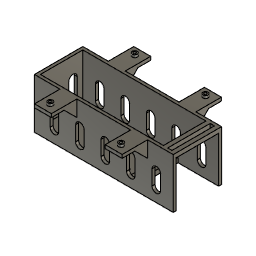
Battery Housing Vertical Slits (Autodesk Fusion 360 design; units mm, degrees)
Autodesk Fusion 360 part; units mm, degrees
sketch "Sketch1" plane through (0, 0, 0) normal (1, 0, 0) x (0, 1, 0)
  line L0 (0, 0) -> (57, 0)
  line L1 (57, 0) -> (57, 57)
  line L2 (57, 57) -> (0, 57)
  line L3 (0, 57) -> (0, 0)
  line L4 (3.5, 57) -> (53.5, 57)
  line L5 (53.5, 57) -> (53.5, 3.5)
  line L6 (53.5, 3.5) -> (3.5, 3.5)
  line L7 (3.5, 3.5) -> (3.5, 57)
  dimension "d1" = 57
  dimension "d2" = 57
  dimension "d3" = 3.5
  dimension "d4" = 3.5
  dimension "d5" = 3.5
  constraint horizontal L0
  constraint vertical L1
  constraint horizontal L2
  constraint vertical L3
  constraint coincident L0.start L3.end
  constraint horizontal L4
  constraint vertical L5
  constraint horizontal L6
  constraint vertical L7
  constraint coincident L2 L4.start
  measures "d1" distance of L0.start L0.end
  measures "d2" distance of L0.start L2.end
  measures "d3" distance of L1 L5
  measures "d4" distance of L3 L7
  measures "d5" distance of L0 L6
extrude "Extrude1" add sketch "Sketch1" along normal blind 160 contours L0 L1 L2 L3 L5 L6 L7
sketch "Sketch2" plane through (0, 0, 0) normal (-1, 0, 0) x (0, -1, 0)
  line L0 (-3.5, 57) -> (-3.5, 3.5)
  line L1 (-3.5, 3.5) -> (-53.5, 3.5)
  line L2 (-53.5, 3.5) -> (-53.5, 57)
  line L3 (-53.5, 57) -> (-57, 57)
  line L4 (-57, 57) -> (-57, 0)
  line L5 (-57, 0) -> (0, 0)
  line L6 (0, 0) -> (0, 57)
  line L7 (0, 57) -> (-3.5, 57)
  line L8 (-57, 57) -> (0, 57)
  line L9 (0, 57) -> (0, 0)
  line L10 (0, 0) -> (-57, 0)
  line L11 (-57, 0) -> (-57, 57)
  constraint horizontal L8
  constraint vertical L9
  constraint horizontal L10
  constraint vertical L11
  constraint coincident L5.end L6.start
  constraint coincident L3.end L4.start
extrude "Extrude2" add sketch "Sketch2" along normal blind 3.5
ref_plane "WorkPlane1" through (78.25, 28.5, 57) normal (0, 0, 1) x (0, -1, 0)
sketch "Sketch4" plane through (0, 0, 57) normal (0, 0, 1) x (1, 0, 0)
  circle A0 centre (36.5, 78.25) radius 1.5
  circle A1 centre (119.8, 78.25) radius 1.5
  circle A2 centre (36.5, -21.25) radius 1.5
  circle A3 centre (119.8, -21.25) radius 1.5
  line L0 (-3.5, 57) -> (160, 57)
  line L1 (26.5, 0) -> (46.5, 0)
  line L2 (46.5, 0) -> (46.5, -30)
  line L3 (46.5, -30) -> (26.5, -30)
  line L4 (26.5, -30) -> (26.5, 0)
  line L5 (109.8, 0) -> (129.8, 0)
  line L6 (129.8, 0) -> (129.8, -30)
  line L7 (129.8, -30) -> (109.8, -30)
  line L8 (109.8, -30) -> (109.8, 0)
  line L9 (109.8, 57) -> (129.8, 57)
  line L10 (129.8, 57) -> (129.8, 87)
  line L11 (129.8, 87) -> (109.8, 87)
  line L12 (109.8, 87) -> (109.8, 57)
  line L13 (26.5, 87) -> (46.5, 87)
  line L14 (46.5, 87) -> (46.5, 57)
  line L15 (46.5, 57) -> (26.5, 57)
  line L16 (26.5, 57) -> (26.5, 87)
  line L17 (-3.5, 57) -> (-3.5, 54.574)
  line L18 (-3.5, 0) -> (-3.5, 57)
  point P0 (-3.5, 57)
  dimension "d27" = 3
  dimension "d29" = 3
  dimension "d31" = 3
  dimension "d33" = 3
  dimension "d38" = 21.25
  dimension "d39" = 10
  dimension "d40" = 10
  dimension "d41" = 20
  dimension "d42" = 30
  dimension "d43" = 20
  dimension "d44" = 30
  dimension "d45" = 10
  dimension "d46" = 10
  dimension "d47" = 21.25
  dimension "d51" = 30
  dimension "d52" = 20
  dimension "d53" = 30
  dimension "d54" = 20
  dimension "d186" = 63.3
  dimension "d187" = 63.3
  dimension "d188" = 103.3
  dimension "d189" = 163.5
  dimension "d190" = 30
  dimension "d191" = 30
  constraint horizontal L1
  constraint vertical L2
  constraint horizontal L3
  constraint vertical L4
  constraint horizontal L5
  constraint vertical L6
  constraint horizontal L7
  constraint vertical L8
  constraint horizontal L9
  constraint vertical L10
  constraint horizontal L11
  constraint vertical L12
  constraint horizontal L13
  constraint vertical L14
  constraint horizontal L15
  constraint vertical L16
  constraint coincident P0 L0.start
  constraint perpendicular L0 L17
  measures "d27" diameter of A0
  measures "d29" diameter of A1
  measures "d31" diameter of A2
  measures "d33" diameter of A3
  measures "d38" distance of A0.centre L0
  measures "d39" distance of A3.centre L8
  measures "d40" distance of A2.centre L4
  measures "d41" distance of L9.start L9.end
  measures "d42" distance of L9.start L11.end
  measures "d43" distance of L13.start L13.end
  measures "d44" distance of L13.start L15.end
  measures "d45" distance of A1.centre L12
  measures "d46" distance of A0.centre L16
  measures "d47" distance of A0.centre L15
  measures "d51" distance of L5.end L6.end
  measures "d52" distance of L6.end L7.end
  measures "d53" distance of L1.end L2.end
  measures "d54" distance of L2.end L3.end
  measures "d186" distance of L12 L14
  measures "d187" distance of L2 L8
  measures "d188" distance of L10 L16
  measures "d189" distance of P0 L0.end
  measures "d190" distance of L16 L18
  measures "d191" distance of L4 L18
extrude "Extrude4" add sketch "Sketch4" against normal blind 4
sketch "Sketch5" plane through (129.8, 0, 0) normal (1, 0, 0) x (0, 1, 0)
  line L0 (0, 57) -> (-30, 57)
  line L1 (-30, 57) -> (-30, 53)
  line L2 (-30, 53) -> (0, 53)
  line L3 (0, 53) -> (0, 57)
  line L4 (0, 53) -> (-15, 53)
  line L5 (-15, 53) -> (0, 38)
  line L6 (0, 38) -> (0, 53)
  dimension "d55" = 45
  constraint coincident L2.end L3.start
  constraint midpoint L2 L4.end
  constraint perpendicular L4 L6
  measures "d55" angle of L4 L5
extrude "Extrude5" add sketch "Sketch5" against normal blind 2 contours L2 L4 L5 L6
sketch "Sketch6" plane through (129.8, 0, 0) normal (1, 0, 0) x (0, 1, 0)
  line L0 (87, 57) -> (57, 57)
  line L1 (57, 57) -> (57, 53)
  line L2 (57, 53) -> (87, 53)
  line L3 (87, 53) -> (87, 57)
  line L4 (57, 53) -> (72, 53)
  line L5 (72, 53) -> (57, 38)
  line L6 (57, 38) -> (57, 53)
  dimension "d58" = 45
  constraint coincident L1.end L2.start
  constraint midpoint L2 L4.end
  constraint perpendicular L2 L6
  measures "d58" angle of L4 L5
extrude "Extrude6" add sketch "Sketch6" against normal blind 2 contours L2 L4 L5 L6
sketch "Sketch7" plane through (109.8, 0, 0) normal (-1, 0, 0) x (0, -1, 0)
  line L0 (-57, 57) -> (-87, 57)
  line L1 (-87, 57) -> (-87, 53)
  line L2 (-87, 53) -> (-57, 53)
  line L3 (-57, 53) -> (-57, 57)
  line L4 (-57, 53) -> (-72, 53)
  line L5 (-72, 53) -> (-57, 38)
  line L6 (-57, 38) -> (-57, 53)
  dimension "d61" = 45
  constraint coincident L2.end L3.start
  constraint midpoint L2 L4.end
  constraint perpendicular L4 L6
  measures "d61" angle of L4 L5
extrude "Extrude7" add sketch "Sketch7" against normal blind 2 contours L2 L4 L5 L6
sketch "Sketch8" plane through (109.8, 0, 0) normal (-1, 0, 0) x (0, -1, 0)
  line L0 (30, 57) -> (0, 57)
  line L1 (0, 57) -> (0, 53)
  line L2 (0, 53) -> (30, 53)
  line L3 (30, 53) -> (30, 57)
  line L4 (0, 53) -> (15, 53)
  line L5 (15, 53) -> (0, 38)
  line L6 (0, 38) -> (0, 53)
  dimension "d64" = 45
  constraint coincident L1.end L2.start
  constraint midpoint L2 L4.end
  constraint perpendicular L4 L6
  measures "d64" angle of L4 L5
extrude "Extrude8" add sketch "Sketch8" against normal blind 2 contours L2 L4 L5 L6
sketch "Sketch9" plane through (46.5, 0, 0) normal (1, 0, 0) x (0, 1, 0)
  line L0 (0, 57) -> (-30, 57)
  line L1 (-30, 57) -> (-30, 53)
  line L2 (-30, 53) -> (0, 53)
  line L3 (0, 53) -> (0, 57)
  line L4 (0, 53) -> (-15, 53)
  line L5 (-15, 53) -> (0, 38)
  line L6 (0, 38) -> (0, 53)
  dimension "d67" = 45
  constraint coincident L2.end L3.start
  constraint midpoint L2 L4.end
  constraint perpendicular L4 L6
  measures "d67" angle of L4 L5
extrude "Extrude9" add sketch "Sketch9" against normal blind 2 contours L2 L4 L5 L6
sketch "Sketch10" plane through (26.5, 0, 0) normal (-1, 0, 0) x (0, -1, 0)
  line L0 (30, 57) -> (0, 57)
  line L1 (0, 57) -> (0, 53)
  line L2 (0, 53) -> (30, 53)
  line L3 (30, 53) -> (30, 57)
  line L4 (0, 53) -> (15, 53)
  line L5 (15, 53) -> (0, 38)
  line L6 (0, 38) -> (0, 53)
  constraint coincident L1.end L2.start
  constraint midpoint L2 L4.end
  constraint perpendicular L4 L6
extrude "Extrude10" add sketch "Sketch10" against normal blind 2 contours L2 L4 L5 L6
sketch "Sketch11" plane through (26.5, 0, 0) normal (-1, 0, 0) x (0, -1, 0)
  line L0 (-57, 57) -> (-87, 57)
  line L1 (-87, 57) -> (-87, 53)
  line L2 (-87, 53) -> (-57, 53)
  line L3 (-57, 53) -> (-57, 57)
  line L4 (-57, 53) -> (-72, 53)
  line L5 (-72, 53) -> (-57, 38)
  line L6 (-57, 38) -> (-57, 53)
  constraint coincident L2.end L3.start
  constraint midpoint L2 L4.end
extrude "Extrude11" add sketch "Sketch11" against normal blind 2 contours L2 L4 L5 L6
sketch "Sketch12" plane through (46.5, 0, 0) normal (1, 0, 0) x (0, 1, 0)
  line L0 (87, 57) -> (57, 57)
  line L1 (57, 57) -> (57, 53)
  line L2 (57, 53) -> (87, 53)
  line L3 (87, 53) -> (87, 57)
  line L4 (57, 53) -> (72, 53)
  line L5 (72, 53) -> (57, 38)
  line L6 (57, 38) -> (57, 53)
  dimension "d74" = 45
  constraint coincident L1.end L2.start
  constraint midpoint L2 L4.end
  constraint perpendicular L4 L6
  measures "d74" angle of L4 L5
extrude "Extrude12" add sketch "Sketch12" against normal blind 2 contours L2 L4 L5 L6
extrude "Extrude20" add 1 faces at (105.5, 38, 0) along direction (0, 0, -1) blind 2
sketch "Sketch23" plane through (0, 0, 3.5) normal (0, 0, 1) x (-1, 0, 0)
  line L0 (0, -53.5) -> (0, -3.5)
  line L1 (0, -3.5) -> (-160, -3.5)
  line L2 (-160, -3.5) -> (-160, -53.5)
  line L3 (-160, -53.5) -> (0, -53.5)
  line L4 (-160, -53.5) -> (-102.25, -53.5)
  line L5 (-102.25, -53.5) -> (-102.25, -3.5)
  line L6 (-102.25, -3.5) -> (-160, -3.5)
  line L7 (-160, -3.5) -> (-160, -53.5)
  constraint horizontal L4
  constraint vertical L5
  constraint horizontal L6
  constraint vertical L7
  constraint coincident L1 L5.end
  constraint coincident L2.end L3.start
extrude "Extrude22" cut sketch "Sketch23" against normal up to surface (5.5 mm away) contours L1 L2 L3 L4 L5 L6 L7
sketch "Sketch28" plane through (0, 0, 57) normal (0, 0, 1) x (-1, 0, 0)
  line L0 (-160, 0) -> (-160, -3.5)
  line L1 (-160, -57) -> (-129.8, -57)
  line L2 (-129.8, -57) -> (-129.8, -87)
  line L3 (-129.8, -87) -> (-109.8, -87)
  line L4 (-109.8, -87) -> (-109.8, -57)
  line L5 (-109.8, -57) -> (-46.5, -57)
  line L6 (-46.5, -57) -> (-46.5, -87)
  line L7 (-46.5, -87) -> (-26.5, -87)
  line L8 (-26.5, -87) -> (-26.5, -57)
  line L9 (-26.5, -57) -> (3.5, -57)
  line L10 (3.5, -57) -> (3.5, 0)
  line L11 (3.5, 0) -> (-26.5, 0)
  line L12 (-26.5, 0) -> (-26.5, 30)
  line L13 (-26.5, 30) -> (-46.5, 30)
  line L14 (-46.5, 30) -> (-46.5, 0)
  line L15 (-46.5, 0) -> (-109.8, 0)
  line L16 (-109.8, 0) -> (-109.8, 30)
  line L17 (-109.8, 30) -> (-129.8, 30)
  line L18 (-129.8, 30) -> (-129.8, 0)
  line L19 (-129.8, 0) -> (-160, 0)
  line L20 (0, -3.5) -> (0, -53.5)
  line L21 (0, -53.5) -> (-160, -53.5)
  line L22 (-160, -3.5) -> (0, -3.5)
  circle A0 centre (-119.8, 21.25) radius 1.5
  circle A1 centre (-36.5, 21.25) radius 1.5
  circle A2 centre (-119.8, -78.25) radius 1.5
  circle A3 centre (-36.5, -78.25) radius 1.5
  circle A4 centre (-36.5, -78.25) radius 1.5
  circle A5 centre (-119.8, -78.25) radius 1.5
  circle A6 centre (-36.5, 21.25) radius 1.5
  circle A7 centre (-119.8, 21.25) radius 1.5
  circle A8 centre (-119.8, 21.25) radius 3
  circle A9 centre (-36.5, 21.25) radius 3
  circle A10 centre (-36.5, -78.25) radius 3
  circle A11 centre (-119.8, -78.25) radius 3
  line L23 (-160, -53.5) -> (-160, -57)
  dimension "d249" = 3
  dimension "d250" = 3
  dimension "d251" = 3
  dimension "d252" = 3
  dimension "d253" = 6
  dimension "d254" = 6
  dimension "d255" = 6
  dimension "d256" = 6
  constraint concentric A3 A4
  constraint concentric A2 A5
  constraint concentric A1 A6
  constraint concentric A0 A7
  constraint concentric A0 A8
  constraint concentric A6 A9
  constraint concentric A4 A10
  constraint concentric A5 A11
  measures "d249" diameter of A4
  measures "d250" diameter of A5
  measures "d251" diameter of A6
  measures "d252" diameter of A7
  measures "d253" diameter of A8
  measures "d254" diameter of A9
  measures "d255" diameter of A10
  measures "d256" diameter of A11
extrude "Extrude27" add sketch "Sketch28" along normal blind 3 contours A8 | A9 | A10 | A11
sketch "Sketch30" plane through (0, 57, 0) normal (0, 1, 0) x (-1, 0, 0)
  line L0 (-46.5, 38) -> (-46.5, 57)
  line L1 (-46.5, 57) -> (-109.8, 57)
  line L2 (-109.8, 57) -> (-109.8, 38)
  line L3 (-109.8, 38) -> (-111.8, 38)
  line L4 (-111.8, 38) -> (-111.8, 53)
  line L5 (-111.8, 53) -> (-127.8, 53)
  line L6 (-127.8, 53) -> (-127.8, 38)
  line L7 (-127.8, 38) -> (-129.8, 38)
  line L8 (-129.8, 38) -> (-129.8, 57)
  line L9 (-129.8, 57) -> (-160, 57)
  line L10 (-160, 57) -> (-160, -2)
  line L11 (-160, -2) -> (3.5, -2)
  line L12 (3.5, -2) -> (3.5, 57)
  line L13 (3.5, 57) -> (-26.5, 57)
  line L14 (-26.5, 57) -> (-26.5, 38)
  line L15 (-26.5, 38) -> (-28.5, 38)
  line L16 (-28.5, 38) -> (-28.5, 53)
  line L17 (-28.5, 53) -> (-44.5, 53)
  line L18 (-44.5, 53) -> (-44.5, 38)
  line L19 (-44.5, 38) -> (-46.5, 38)
  arc A0 (-140, 35) -> (-140, 25) centre (-140, 30) ccw
  arc A1 (-140, 17.5) -> (-140, 7.5) centre (-140, 12.5) ccw
  line L20 (-140, 30) -> (-110, 30)
  line L21 (-105, 30) -> (-85, 30)
  line L22 (-80, 30) -> (-55, 30)
  line L23 (-50, 30) -> (-20, 30)
  line L24 (-140, 12.5) -> (-110, 12.5)
  line L25 (-105, 12.5) -> (-80, 12.5)
  line L26 (-75, 12.5) -> (-55, 12.5)
  line L27 (-145, 30) -> (-145, 12.5)
  line L28 (-135, 30) -> (-135, 12.5)
  line L29 (-115, 30) -> (-115, 12.5)
  line L30 (-105, 30) -> (-105, 12.5)
  line L31 (-75, 30) -> (-75, 12.5)
  line L32 (-85, 30) -> (-85, 12.5)
  line L33 (-45, 30) -> (-45, 12.5)
  line L34 (-55, 30) -> (-55, 12.5)
  line L35 (-25, 30) -> (-25, 12.5)
  line L36 (-15, 30) -> (-15, 12.5)
  arc A2 (-25, 12.5) -> (-15, 12.5) centre (-20, 12.5) ccw
  arc A3 (-15, 30) -> (-25, 30) centre (-20, 30) ccw
  arc A4 (-55, 12.5) -> (-45, 12.5) centre (-50, 12.5) ccw
  arc A5 (-45, 30) -> (-55, 30) centre (-50, 30) ccw
  line L37 (-75, 12.5) -> (-20, 12.5)
  arc A6 (-85, 12.5) -> (-75, 12.5) centre (-80, 12.5) ccw
  arc A7 (-75, 30) -> (-85, 30) centre (-80, 30) ccw
  arc A8 (-105, 30) -> (-115, 30) centre (-110, 30) ccw
  arc A9 (-115, 12.5) -> (-105, 12.5) centre (-110, 12.5) ccw
  line L38 (-140, 12.5) -> (-115, 12.5)
  line L39 (-105, 12.5) -> (-85, 12.5)
  arc A10 (-135, 30) -> (-145, 30) centre (-140, 30) ccw
  arc A11 (-145, 12.5) -> (-135, 12.5) centre (-140, 12.5) ccw
  dimension "d264" = 10
  dimension "d265" = 5
  dimension "d266" = 10
  dimension "d315" = 10
  dimension "d316" = 10
  dimension "d319" = 10
  dimension "d320" = 10
  dimension "d321" = 10
  dimension "d322" = 10
  dimension "d323" = 10
  dimension "d324" = 30
  dimension "d325" = 30
  dimension "d326" = 30
  dimension "d327" = 10
  dimension "d328" = 10
  dimension "d329" = 10
  constraint concentric A0 A10
  constraint concentric A1 A11
  constraint coincident A0.centre L20.start
  constraint horizontal L20
  constraint parallel L20 L21
  constraint parallel L21 L22
  constraint parallel L22 L23
  constraint coincident L23.end A3.centre
  constraint coincident L23.start A5.centre
  constraint coincident L22.start A7.centre
  constraint coincident L20.end A8.centre
  constraint coincident A1.centre L24.start
  constraint horizontal L38
  constraint coincident A2.centre L37.end
  constraint parallel L24 L38
  constraint parallel L25 L38
  constraint parallel L26 L38
  constraint coincident L25.end A6.centre
  constraint coincident L24.end A9.centre
  constraint midpoint A0 L27.start
  constraint midpoint A1 L27.end
  constraint tangent L27 A11
  constraint coincident L20 L28.start
  constraint coincident L24 L28.end
  constraint coincident L20 L29.start
  constraint coincident L24 L29.end
  constraint coincident L22 L31.start
  constraint coincident L23 L33.start
  constraint coincident L33.end L38
  constraint tangent L33 A4
  constraint coincident L23 L35.start
  constraint coincident L35.end L38
  constraint tangent L35 A2
  constraint tangent L36 A2
  constraint perpendicular L36 L38
  constraint collinear L37 L38
  constraint collinear L38 L39
  measures "d264" diameter of A0
  measures "d265" distance of A1.end A1.centre
  measures "d266" diameter of A1
  measures "d315" diameter of A10
  measures "d316" diameter of A11
  measures "d319" diameter of A3
  measures "d320" diameter of A5
  measures "d321" diameter of A7
  measures "d322" diameter of A8
  measures "d323" diameter of A2
  measures "d324" distance of A1.centre L24.end
  measures "d325" distance of L24.end L25.end
  measures "d326" distance of L25.end A4.centre
  measures "d327" diameter of A4
  measures "d328" diameter of A6
  measures "d329" diameter of A9
extrude "Extrude28" cut sketch "Sketch30" against normal up to surface (57 mm away) contours A0 A1 L27 L28 A10 A11 | L29 L30 A8 A9 | L31 L32 A6 A7 | L33 L34 A5 L37 | A4 L37 | L35 L36 A2 A3
sketch "Sketch31" plane through (-3.5, 0, 0) normal (-1, 0, 0) x (0, -1, 0)
  line L0 (0, -2) -> (0, 57)
  line L1 (0, 57) -> (-57, 57)
  line L2 (-57, 57) -> (-57, -2)
  line L3 (-57, -2) -> (0, -2)
  line L4 (-37, 33) -> (-37, 12.5)
  line L5 (-42, 7.5) -> (-47, 7.5)
  line L6 (-47, 12.5) -> (-47, 33)
  line L7 (-10, 33) -> (-10, 12.5)
  line L8 (-20, 12.5) -> (-20, 33)
  line L9 (-42, 7.5) -> (-42, 12.5)
  line L10 (-42, 38) -> (-42, 33)
  line L11 (-15, 7.5) -> (-15, 12.5)
  line L12 (-15, 38) -> (-15, 33)
  arc A0 (-37, 33) -> (-47, 33) centre (-42, 33) ccw
  arc A1 (-47, 12.5) -> (-37, 12.5) centre (-42, 12.5) ccw
  arc A2 (-20, 12.5) -> (-10, 12.5) centre (-15, 12.5) ccw
  arc A3 (-10, 33) -> (-20, 33) centre (-15, 33) ccw
  dimension "d272" = 10
  dimension "d273" = 9.5
  dimension "d278" = 10
  dimension "d279" = 5
  dimension "d280" = 10
  dimension "d281" = 5
  dimension "d282" = 10
  dimension "d283" = 5
  dimension "d284" = 10
  dimension "d285" = 5
  dimension "d286" = 10
  constraint vertical L4
  constraint horizontal L5
  constraint vertical L6
  constraint vertical L7
  constraint vertical L8
  constraint perpendicular L5 L9
  constraint coincident L9.end A1.centre
  constraint coincident L10.end A0.centre
  constraint coincident L11.end A2.centre
  constraint coincident L12.end A3.centre
  measures "d272" distance of L2 L6
  measures "d273" distance of L3 L5
  measures "d278" distance of L0 L7
  measures "d279" distance of L5.start L9.end
  measures "d280" diameter of A1
  measures "d281" distance of L10.start L10.end
  measures "d282" diameter of A0
  measures "d283" distance of L11.start L11.end
  measures "d284" diameter of A2
  measures "d285" distance of L12.start L12.end
  measures "d286" diameter of A3
extrude "Extrude29" cut sketch "Sketch31" against normal up to surface (3.5 mm away) contours L4 L6 A0 A1 | L7 L8 A2 A3
sketch "Sketch32" plane through (0, 0, 3.5) normal (0, 0, 1) x (-1, 0, 0)
  line L0 (-102.25, -3.5) -> (-102.25, -53.5)
  line L1 (-102.25, -53.5) -> (0, -53.5)
  line L2 (0, -53.5) -> (0, -3.5)
  line L3 (0, -3.5) -> (-102.25, -3.5)
  circle A0 centre (-94.25, -11.5) radius 1.5
  circle A1 centre (-94.25, -45.5) radius 1.5
  circle A2 centre (-60.25, -11.5) radius 1.5
  circle A3 centre (-60.25, -45.5) radius 1.5
  dimension "d289" = 3
  dimension "d290" = 3
  dimension "d291" = 8
  dimension "d292" = 8
  dimension "d293" = 34
  dimension "d294" = 8
  dimension "d300" = 3
  dimension "d301" = 3
  dimension "d302" = 34
  dimension "d303" = 34
  dimension "d304" = 8
  dimension "d305" = 8
  measures "d289" diameter of A0
  measures "d290" diameter of A1
  measures "d291" distance of L0 A1.centre
  measures "d292" distance of L0 A0.centre
  measures "d293" distance of A0.centre A1.centre
  measures "d294" distance of L3 A0.centre
  measures "d300" diameter of A2
  measures "d301" diameter of A3
  measures "d302" distance of A1.centre A3.centre
  measures "d303" distance of A0.centre A2.centre
  measures "d304" distance of L3 A2.centre
  measures "d305" distance of L1 A3.centre
hole "Hole1" at (94.25, 11.5, 3.5) at (94.25, 45.5, 3.5) at (60.25, 45.5, 3.5) at (60.25, 11.5, 3.5) direction (0, 0, -1) diameter 3 depth 20 tip angle 180 counterbore diameter 5 counterbore depth 2
sketch "Sketch33" plane through (0, 0, -2) normal (0, 0, -1) x (1, 0, 0)
  circle A0 centre (60.25, -45.5) radius 1.5
  circle A1 centre (94.25, -11.5) radius 1.5
  circle A2 centre (94.25, -45.5) radius 1.5
  circle A3 centre (60.25, -11.5) radius 1.5
  line L0 (160, -53.5) -> (102.25, -53.5)
  line L1 (102.25, -53.5) -> (102.25, -3.5)
  line L2 (102.25, -3.5) -> (160, -3.5)
  line L3 (160, -3.5) -> (160, 0)
  line L4 (160, 0) -> (-3.5, 0)
  line L5 (-3.5, 0) -> (-3.5, -57)
  line L6 (-3.5, -57) -> (160, -57)
  line L7 (160, -57) -> (160, -53.5)
  line L8 (102.25, -53.5) -> (107.25, -53.5)
  line L9 (107.25, -53.5) -> (107.25, -3.5)
  line L10 (107.25, -3.5) -> (102.25, -3.5)
  line L11 (102.25, -3.5) -> (102.25, -53.5)
  line L12 (107.25, -53.5) -> (112.25, -53.5)
  line L13 (112.25, -53.5) -> (112.25, -3.5)
  line L14 (112.25, -3.5) -> (107.25, -3.5)
  line L15 (107.25, -3.5) -> (107.25, -53.5)
  dimension "d306" = 5
  dimension "d307" = 5
  constraint horizontal L8
  constraint vertical L9
  constraint horizontal L10
  constraint vertical L11
  constraint coincident L0.end L1.start
  constraint horizontal L12
  constraint vertical L13
  constraint horizontal L14
  constraint vertical L15
  measures "d306" distance of L0.end L8.end
  measures "d307" distance of L8.end L12.end
extrude "Extrude30" add sketch "Sketch33" against normal up to surface (5.5 mm away) contours L0 L2 L9 L12 L13 L14 L15
sketch "Sketch34" plane through (0, 0, 57) normal (0, 0, 1) x (-1, 0, 0)
  circle A0 centre (-36.5, 21.25) radius 3
  circle A1 centre (-36.5, -78.25) radius 3
  circle A2 centre (-119.8, 21.25) radius 3
  circle A3 centre (-119.8, -78.25) radius 3
  line L0 (3.5, 0) -> (-26.5, 0)
  line L1 (-26.5, 0) -> (-26.5, 30)
  line L2 (-26.5, 30) -> (-46.5, 30)
  line L3 (-46.5, 30) -> (-46.5, 0)
  line L4 (-46.5, 0) -> (-109.8, 0)
  line L5 (-109.8, 0) -> (-109.8, 30)
  line L6 (-109.8, 30) -> (-129.8, 30)
  line L7 (-129.8, 30) -> (-129.8, 0)
  line L8 (-129.8, 0) -> (-160, 0)
  line L9 (-160, 0) -> (-160, -3.5)
  line L10 (-160, -3.5) -> (0, -3.5)
  line L11 (0, -3.5) -> (0, -53.5)
  line L12 (0, -53.5) -> (-160, -53.5)
  line L13 (-160, -53.5) -> (-160, -57)
  line L14 (-160, -57) -> (-129.8, -57)
  line L15 (-129.8, -57) -> (-129.8, -87)
  line L16 (-129.8, -87) -> (-109.8, -87)
  line L17 (-109.8, -87) -> (-109.8, -57)
  line L18 (-109.8, -57) -> (-46.5, -57)
  line L19 (-46.5, -57) -> (-46.5, -87)
  line L20 (-46.5, -87) -> (-26.5, -87)
  line L21 (-26.5, -87) -> (-26.5, -57)
  line L22 (-26.5, -57) -> (3.5, -57)
  line L23 (3.5, -57) -> (3.5, 0)
  line L24 (-160, -3.5) -> (-155, -3.5)
  line L25 (-155, -3.5) -> (-155, -53.5)
  line L26 (-155, -53.5) -> (-160, -53.5)
  line L27 (-160, -53.5) -> (-160, -3.5)
  line L28 (-155, -3.5) -> (-150, -3.5)
  line L29 (-150, -3.5) -> (-150, -53.5)
  line L30 (-150, -53.5) -> (-155, -53.5)
  line L31 (-155, -53.5) -> (-155, -3.5)
  line L32 (-150, -3.5) -> (-145, -3.5)
  line L33 (-145, -3.5) -> (-145, -53.5)
  line L34 (-145, -53.5) -> (-150, -53.5)
  line L35 (-150, -53.5) -> (-150, -3.5)
  dimension "d310" = 5
  dimension "d311" = 5
  dimension "d312" = 5
  constraint horizontal L24
  constraint vertical L25
  constraint horizontal L26
  constraint vertical L27
  constraint coincident L9.end L10.start
  constraint horizontal L28
  constraint vertical L29
  constraint horizontal L30
  constraint vertical L31
  constraint horizontal L32
  constraint vertical L33
  constraint horizontal L34
  constraint vertical L35
  measures "d310" distance of L9.end L24.end
  measures "d311" distance of L24.end L28.end
  measures "d312" distance of L28.end L32.end
extrude "Extrude31" add sketch "Sketch34" against normal blind 5 contours L10 L12 L24 L25 L26 L27 L31 | L10 L12 L29 L32 L33 L34 L35
